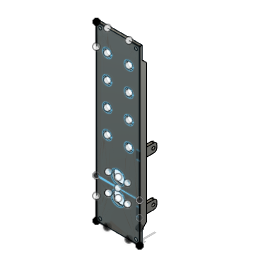
Midi-8x Trigger (Autodesk Fusion 360 design; units mm, degrees)
Autodesk Fusion 360 part; units mm, degrees
note: some values were not read from the file. Set by a fixed rule: which sketch regions a step uses.
sketch "Sketch1" plane through (0, 0, 0) normal (0, 0, 1) x (1, 0, 0)
  line L0 (-8.0882, 5) -> (41.9118, 5)
  line L1 (41.9118, 5) -> (41.9118, 205)
  line L2 (41.9118, 205) -> (-8.0882, 205)
  line L3 (-8.0882, 205) -> (-8.0882, 5)
  line L4 (-8.0882, 205) -> (-3.8456, 200.7574)
  line L5 (-8.0882, 205) -> (6, 205) construction
  line L6 (-8.0882, 5) -> (-3.8456, 9.2426)
  line L7 (-8.0882, 5) -> (6, 5) construction
  line L8 (16.9118, 205) -> (16.9118, 5)
  circle A0 centre (-3.8456, 200.7574) radius 1.75
  circle A1 centre (-3.8456, 9.2426) radius 1.75
  circle A2 centre (37.6691, 200.7574) radius 1.75
  circle A3 centre (37.6691, 9.2426) radius 1.75
  dimension "d1" = 200
  dimension "d2" = 50
  dimension "d3" = 6
  dimension "d4" = 45
  dimension "d5" = 45
  dimension "d6" = 6
  dimension "d7" = 3.5
  dimension "d8" = 3.5
  constraint horizontal L0
  constraint vertical L1
  constraint horizontal L2
  constraint vertical L3
  constraint horizontal L5
  constraint horizontal L7
  constraint midpoint L2 L8.start
  constraint midpoint L0 L8.end
  constraint coincident L4.end A0.centre
  constraint coincident L6.end A1.centre
  constraint symmetric L8 A0 A2
  constraint symmetric L8 A1 A3
  measures "d1" distance of L0.start L2.end
  measures "d2" distance of L1.end L2.end
  measures "d3" distance of L2.end L4.end
  measures "d4" angle of L4 L5
  measures "d5" angle of L6 L7
  measures "d6" distance of L0.start L6.end
  measures "d7" diameter of A0
  measures "d8" diameter of A1
extrude "Extrude1" add sketch "Sketch1" along normal blind 3
sketch "Sketch2" plane through (0, 0, 3) normal (0, 0, 1) x (1, 0, 0)
  circle A0 centre (-3.8456, 200.7574) radius 1.75
  circle A1 centre (37.6691, 9.2426) radius 1.75
  circle A2 centre (-3.8456, 9.2426) radius 1.75
  circle A3 centre (37.6691, 200.7574) radius 1.75
  line L0 (-8.0882, 205) -> (-8.0882, 5)
  line L1 (-8.0882, 5) -> (41.9118, 5)
  line L2 (41.9118, 5) -> (41.9118, 205)
  line L3 (41.9118, 205) -> (-8.0882, 205)
  line L4 (41.9118, 5) -> (29.4118, 5)
  line L5 (29.4118, 205) -> (41.9118, 205)
  line L6 (41.9118, 205) -> (41.9118, 5)
  line L7 (-8.0882, 5) -> (4.4118, 5)
  line L8 (4.4118, 205) -> (-8.0882, 205)
  line L9 (-8.0882, 205) -> (-8.0882, 5)
  line L10 (-8.0882, 205) -> (-8.0882, 180)
  line L11 (-8.0882, 5) -> (-8.0882, 30)
  circle A4 centre (4.4118, 180) radius 4.75
  circle A5 centre (4.4118, 152.5) radius 4.75
  circle A6 centre (4.4118, 125) radius 4.75
  circle A7 centre (4.4118, 97.5) radius 4.75
  circle A8 centre (29.4118, 152.5) radius 4.75
  circle A9 centre (29.4118, 125) radius 4.75
  circle A10 centre (29.4118, 180) radius 4.75
  circle A11 centre (29.4118, 97.5) radius 4.75
  circle A12 centre (16.9118, 61.25) radius 7.75
  circle A13 centre (5.8118, 61.25) radius 1.6
  circle A14 centre (28.0118, 61.25) radius 1.6
  line L12 (16.9118, 50.625) -> (-8.0882, 50.625)
  line L13 (-8.0882, 50.625) -> (41.9118, 50.625)
  circle A15 centre (16.9118, 40) radius 7.75
  circle A16 centre (28.0118, 40) radius 1.6
  circle A17 centre (5.8118, 40) radius 1.6
  point P0 (28.0118, 40)
  point P1 (5.8118, 40)
  dimension "d11" = 12.5
  dimension "d12" = 200
  dimension "d13" = 12.5
  dimension "d14" = 200
  dimension "d15" = 9.5
  dimension "d17" = 27.5
  dimension "d18" = 9.5
  dimension "d19" = 27.5
  dimension "d20" = 9.5
  dimension "d21" = 27.5
  dimension "d22" = 9.5
  dimension "d23" = 92.5
  dimension "d25" = 15.5
  dimension "d26" = 11.1
  dimension "d27" = 3.2
  constraint horizontal L4
  constraint horizontal L5
  constraint vertical L6
  constraint coincident L1.end L2.start
  constraint horizontal L7
  constraint horizontal L8
  constraint vertical L9
  constraint coincident L0.end L1.start
  constraint coincident L0.start L3.end
  constraint coincident L9 L10.end
  constraint perpendicular L8 L10
  constraint coincident L9 L11.end
  constraint perpendicular L1 L11
  constraint coincident L0 L12.end
  constraint perpendicular L0 L12
  constraint coincident L2 L13.end
  constraint perpendicular L2 L13
  constraint symmetric A12 L13 A15
  constraint symmetric A13.centre L13 P1
  constraint symmetric A14.centre L13 P0
  constraint symmetric A13 L13 A17
  constraint symmetric A14 L13 A16
  measures "d11" distance of L1.end L4.end
  measures "d12" distance of L1.end L2.end
  measures "d13" distance of L0.end L7.end
  measures "d14" distance of L0.end L0.start
  measures "d15" diameter of A4
  measures "d17" distance of A4.centre A5.centre
  measures "d18" diameter of A5
  measures "d19" distance of A5.centre A6.centre
  measures "d20" diameter of A6
  measures "d21" distance of A6.centre A7.centre
  measures "d22" diameter of A7
  measures "d23" distance of L7.end A7.centre
  measures "d25" diameter of A12
  measures "d26" distance of A12.centre A13.centre
  measures "d27" diameter of A13
extrude "Extrude2" cut sketch "Sketch2" against normal blind 3 contours A4 | A5 | A6 | A7 | A8 | A9 | A10 | A11 | A12 | A13 | A14
sketch "Sketch3" plane through (0, 0, 0) normal (0, 0, -1) x (-1, 0, 0)
  circle A0 centre (-4.4118, 152.5) radius 4.75
  circle A1 centre (-29.4118, 97.5) radius 4.75
  circle A2 centre (-16.9118, 61.25) radius 7.75
  circle A3 centre (-4.4118, 97.5) radius 4.75
  circle A4 centre (-29.4118, 152.5) radius 4.75
  circle A5 centre (-4.4118, 180) radius 4.75
  circle A6 centre (-29.4118, 125) radius 4.75
  circle A7 centre (-28.0118, 61.25) radius 1.6
  circle A8 centre (-5.8118, 61.25) radius 1.6
  circle A9 centre (-4.4118, 125) radius 4.75
  circle A10 centre (-29.4118, 180) radius 4.75
  circle A11 centre (3.8456, 200.7574) radius 1.75
  circle A12 centre (-37.6691, 9.2426) radius 1.75
  circle A13 centre (3.8456, 9.2426) radius 1.75
  circle A14 centre (-37.6691, 200.7574) radius 1.75
  line L0 (8.0882, 5) -> (8.0882, 205)
  line L1 (8.0882, 205) -> (-41.9118, 205)
  line L2 (-41.9118, 205) -> (-41.9118, 5)
  line L3 (-41.9118, 5) -> (8.0882, 5)
  line L4 (-41.9118, 205) -> (-38.9118, 205)
  line L5 (-38.9118, 205) -> (-38.9118, 190)
  line L6 (-38.9118, 190) -> (-41.9118, 190)
  line L7 (-41.9118, 190) -> (-41.9118, 205)
  line L8 (-16.9118, 205) -> (-16.9118, 5)
  line L9 (8.0882, 205) -> (5.0882, 205)
  line L10 (5.0882, 205) -> (5.0882, 190)
  line L11 (5.0882, 190) -> (8.0882, 190)
  line L12 (8.0882, 190) -> (8.0882, 205)
  line L13 (-41.9118, 5) -> (-38.9118, 5)
  line L14 (-38.9118, 5) -> (-38.9118, 20)
  line L15 (-38.9118, 20) -> (-41.9118, 20)
  line L16 (-41.9118, 20) -> (-41.9118, 5)
  line L17 (8.0882, 5) -> (5.0882, 5)
  line L18 (5.0882, 5) -> (5.0882, 20)
  line L19 (5.0882, 20) -> (8.0882, 20)
  line L20 (8.0882, 20) -> (8.0882, 5)
  line L21 (-41.9118, 190) -> (-38.9118, 190)
  line L22 (-38.9118, 190) -> (-38.9118, 20)
  line L23 (-38.9118, 20) -> (-41.9118, 20)
  line L24 (-41.9118, 20) -> (-41.9118, 190)
  line L25 (5.0882, 190) -> (8.0882, 190)
  line L26 (8.0882, 190) -> (8.0882, 20)
  line L27 (8.0882, 20) -> (5.0882, 20)
  line L28 (5.0882, 20) -> (5.0882, 190)
  dimension "d30" = 3
  dimension "d31" = 15
  dimension "d32" = 3
  dimension "d33" = 15
  dimension "d34" = 3
  dimension "d35" = 15
  dimension "d36" = 3
  dimension "d37" = 15
  constraint horizontal L4
  constraint vertical L5
  constraint horizontal L6
  constraint vertical L7
  constraint coincident L1.end L2.start
  constraint midpoint L1 L8.start
  constraint midpoint L3 L8.end
  constraint horizontal L9
  constraint vertical L10
  constraint horizontal L11
  constraint vertical L12
  constraint coincident L0.end L1.start
  constraint horizontal L13
  constraint vertical L14
  constraint horizontal L15
  constraint vertical L16
  constraint coincident L2.end L3.start
  constraint horizontal L17
  constraint vertical L18
  constraint horizontal L19
  constraint vertical L20
  constraint coincident L0.start L3.end
  constraint horizontal L21
  constraint vertical L22
  constraint horizontal L23
  constraint vertical L24
  constraint horizontal L25
  constraint vertical L26
  constraint horizontal L27
  constraint vertical L28
  measures "d30" distance of L1.end L4.end
  measures "d31" distance of L1.end L6.end
  measures "d32" distance of L0.end L9.end
  measures "d33" distance of L0.end L11.end
  measures "d34" distance of L2.end L13.end
  measures "d35" distance of L2.end L15.end
  measures "d36" distance of L0.start L17.end
  measures "d37" distance of L0.start L19.end
extrude "Extrude3" add sketch "Sketch3" along normal blind 5 contours L0 L11 L19 L25 L26 L27 L28 | L2 L6 L15 L21 L22 L23 L24
sketch "Sketch4" plane through (0, 0, 0) normal (0, 0, -1) x (-1, 0, 0)
  circle A0 centre (-37.6691, 200.7574) radius 1.75
  circle A1 centre (3.8456, 9.2426) radius 1.75
  circle A2 centre (-37.6691, 9.2426) radius 1.75
  circle A3 centre (3.8456, 200.7574) radius 1.75
  circle A4 centre (-29.4118, 180) radius 4.75
  circle A5 centre (-4.4118, 125) radius 4.75
  circle A6 centre (-5.8118, 61.25) radius 1.6
  circle A7 centre (-28.0118, 61.25) radius 1.6
  circle A8 centre (-29.4118, 125) radius 4.75
  circle A9 centre (-4.4118, 180) radius 4.75
  circle A10 centre (-29.4118, 152.5) radius 4.75
  circle A11 centre (-4.4118, 97.5) radius 4.75
  circle A12 centre (-16.9118, 61.25) radius 7.75
  circle A13 centre (-29.4118, 97.5) radius 4.75
  circle A14 centre (-4.4118, 152.5) radius 4.75
  line L0 (-41.9118, 190) -> (-38.9118, 190)
  line L1 (-38.9118, 190) -> (-38.9118, 20)
  line L2 (-38.9118, 20) -> (-41.9118, 20)
  line L3 (-41.9118, 20) -> (-41.9118, 5)
  line L4 (-41.9118, 5) -> (8.0882, 5)
  line L5 (8.0882, 5) -> (8.0882, 20)
  line L6 (8.0882, 20) -> (5.0882, 20)
  line L7 (5.0882, 20) -> (5.0882, 190)
  line L8 (5.0882, 190) -> (8.0882, 190)
  line L9 (8.0882, 190) -> (8.0882, 205)
  line L10 (8.0882, 205) -> (-41.9118, 205)
  line L11 (-41.9118, 205) -> (-41.9118, 190)
  line L12 (-38.9118, 20) -> (-38.9118, 30)
  line L13 (-38.9118, 30) -> (-35.9118, 30)
  line L14 (-35.9118, 30) -> (-35.9118, 40)
  line L15 (-35.9118, 40) -> (-38.9118, 40)
  line L16 (-38.9118, 40) -> (-38.9118, 30)
  line L17 (-38.9118, 40) -> (-38.9118, 87)
  line L18 (-38.9118, 87) -> (-35.9118, 87)
  line L19 (-35.9118, 87) -> (-35.9118, 97)
  line L20 (-35.9118, 97) -> (-38.9118, 97)
  line L21 (-38.9118, 97) -> (-38.9118, 87)
  dimension "d40" = 3
  dimension "d41" = 10
  dimension "d42" = 47
  dimension "d43" = 3
  dimension "d44" = 10
  constraint coincident L1.end L2.start
  constraint coincident L1 L12.end
  constraint perpendicular L2 L12
  constraint horizontal L13
  constraint vertical L14
  constraint horizontal L15
  constraint vertical L16
  constraint perpendicular L15 L17
  constraint horizontal L18
  constraint vertical L19
  constraint horizontal L20
  constraint vertical L21
  measures "d40" distance of L12.end L13.end
  measures "d41" distance of L12.end L15.end
  measures "d42" distance of L15.end L17.end
  measures "d43" distance of L17.end L18.end
  measures "d44" distance of L17.end L20.end
extrude "Extrude4" add sketch "Sketch4" along normal blind 20 contours L1 L18 L19 L20 L21 | L1 L13 L14 L15 L16
fillet "Fillet1" radius 3.5 4 edges at (37.4118, 87, -20) (37.4118, 97, -20) (37.4118, 30, -20) (37.4118, 40, -20)
chamfer "Chamfer1" distance 5 angle 45 2 edges at (40.4118, 20, -5) (-6.5882, 20, -5)
chamfer "Chamfer2" distance 5 angle 45 2 edges at (-6.5882, 190, -5) (40.4118, 190, -5)
sketch "Sketch5" plane through (35.9118, 0, 0) normal (-1, 0, 0) x (0, 0, 1)
  arc A0 (-16.5, 97) -> (-20, 93.5) centre (-16.5, 93.5) ccw
  line L0 (-20, 93.5) -> (-20, 90.5)
  arc A1 (-20, 90.5) -> (-16.5, 87) centre (-16.5, 90.5) ccw
  line L1 (-16.5, 87) -> (0, 87)
  line L2 (0, 87) -> (0, 97)
  line L3 (0, 97) -> (-16.5, 97)
  line L4 (-20, 92) -> (-16, 92)
  circle A2 centre (-16, 92) radius 1.75
  line L5 (-20, 35) -> (-16, 35)
  circle A3 centre (-16, 35) radius 1.75
  dimension "d50" = 4
  dimension "d51" = 3.5
  dimension "d52" = 3.5
  constraint midpoint L0 L4.start
  constraint perpendicular L0 L4
  constraint coincident L4.end A2.centre
  constraint horizontal L5
  constraint coincident L5.end A3.centre
  measures "d50" distance of L4.start L4.end
  measures "d51" diameter of A2
  measures "d52" diameter of A3
extrude "Extrude5" cut sketch "Sketch5" against normal blind 5 contours A2 | A3
extrude "Extrude6" cut sketch "Sketch2" against normal blind 3 contours A15
extrude "Extrude7" cut sketch "Sketch2" against normal blind 3 contours A16 | A17
